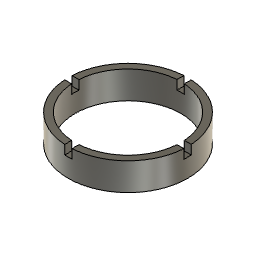
58.4mm-centering v5 (Autodesk Fusion 360 design; units mm, degrees)
Autodesk Fusion 360 part; units mm, degrees
cylinder "CylinderPrimitive1" add diameter 65 height 15 placed x (1, 0, 0) y (0, 1, 0) z (0, 0, 1) at (0, 0, 0)
cylinder "CylinderPrimitive2" cut diameter 57.5 height -15 placed x (1, 0, 0) y (0, 1, 0) z (0, 0, 1) at (0, 0, 15)
sketch "Sketch5" plane through (0, 0, 0) normal (0, 1, 0) x (1, 0, 0)
  line L0 (0, -15) -> (0, 0)
  line L1 (-2, -15) -> (2, -15)
  line L2 (2, -15) -> (2, -10)
  line L3 (2, -10) -> (-2, -10)
  line L4 (-2, -10) -> (-2, -15)
  constraint coincident L0.end origin
  constraint vertical L0
  constraint horizontal L1
  constraint vertical L2
  constraint horizontal L3
  constraint vertical L4
sketch "Sketch6" plane through (0, 0, 0) normal (1, 0, 0) x (0, 1, 0)
  line L0 (0, 15) -> (0, 0)
  line L1 (-2, 15) -> (2, 15)
  line L2 (2, 15) -> (2, 10)
  line L3 (2, 10) -> (-2, 10)
  line L4 (-2, 10) -> (-2, 15)
  constraint coincident L0.end origin
  constraint vertical L0
  constraint horizontal L1
  constraint vertical L2
  constraint horizontal L3
  constraint vertical L4
extrude "Extrude1" cut sketch "Sketch6" along normal through all and the other way through all
extrude "Extrude2" cut sketch "Sketch5" along normal through all and the other way through all
